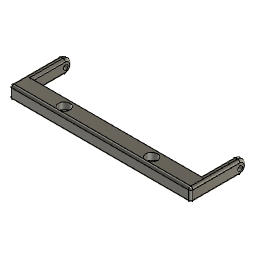
Q.R 2.0 A (Autodesk Fusion 360 design; units mm, degrees)
Autodesk Fusion 360 part; units mm, degrees
note: some values were not read from the file. Chosen so that the rebuilt part matches the saved one: which face or edge a step refers to. Set by a fixed rule: which sketch regions a step uses.
sketch "Sketch5" plane through (0, 0, -8) normal (0, 0, -1) x (1, 0, 0) in component "Arm 2.0 v7"
  arc A0 (69.5, 1.75) -> (68.5, 2.75) centre (68.5, 1.75) ccw
  line L0 (68.5, 2.75) -> (-0.75, 2.75)
  arc A1 (-0.75, 2.75) -> (-2.75, 0.75) centre (-0.75, 0.75) ccw
  line L1 (-2.75, 0.75) -> (-2.75, -47.25)
  arc A2 (-2.75, -47.25) -> (-0.75, -49.25) centre (-0.75, -47.25) ccw
  line L2 (-0.75, -49.25) -> (68.5, -49.25)
  arc A3 (68.5, -49.25) -> (69.5, -48.25) centre (68.5, -48.25) ccw
  line L3 (69.5, -48.25) -> (-1.75, -48.25)
  line L4 (-1.75, -48.25) -> (-1.75, 1.75)
  line L5 (-1.75, 1.75) -> (69.5, 1.75)
  line L6 (0.6613, 2.75) -> (-4.5, 2.75)
  line L7 (-2.75, -0.7377) -> (-2.75, 4.5)
  line L8 (-2.75, 2.75) -> (69.5271, 2.75)
  line L9 (69.5271, 2.75) -> (69.5271, -49.2656)
  line L10 (69.5271, -49.2656) -> (-2.75, -49.2656)
  line L11 (-2.75, -49.2656) -> (-2.75, 2.75)
  line L12 (70.0271, -49.7656) -> (-3.25, -49.7656)
  line L13 (-3.25, -49.7656) -> (-3.25, 3.25)
  line L14 (-3.25, 3.25) -> (70.0271, 3.25)
  line L15 (70.0271, 3.25) -> (70.0271, -49.7656)
  line L16 (73.0271, -52.7656) -> (-6.25, -52.7656)
  line L17 (-6.25, -52.7656) -> (-6.25, 6.25)
  line L18 (-6.25, 6.25) -> (73.0271, 6.25)
  line L19 (73.0271, 6.25) -> (73.0271, -52.7656)
  line L20 (79.5271, -59.2656) -> (-12.75, -59.2656)
  line L21 (-12.75, -59.2656) -> (-12.75, 12.75)
  line L22 (-12.75, 12.75) -> (79.5271, 12.75)
  line L23 (79.5271, 12.75) -> (79.5271, -59.2656)
  line L24 (82.5271, -62.2656) -> (-15.75, -62.2656)
  line L25 (-15.75, -62.2656) -> (-15.75, 15.75)
  line L26 (-15.75, 15.75) -> (82.5271, 15.75)
  line L27 (82.5271, 15.75) -> (82.5271, -62.2656)
  line L28 (-15.75, -3.25) -> (82.5271, -3.25)
  line L29 (-6.25, -3.25) -> (-6.25, 15.75)
  line L30 (70.0271, 3.25) -> (70.0271, 15.75)
  line L31 (73.0271, 6.25) -> (73.0271, 12.75)
  line L32 (-3.25, 3.25) -> (-3.25, 12.75)
  line L33 (73.0271, 12.75) -> (73.0271, 15.75)
  dimension "d13" = -0.5
  dimension "d14" = -3.5
  dimension "d15" = -10
  dimension "d16" = -13
  dimension "d17" = 6
  constraint coincident L0 L6.start
  constraint coincident L1 L7.start
  constraint perpendicular L6 L7
  constraint horizontal L8
  constraint vertical L9
  constraint horizontal L10
  constraint vertical L11
  constraint coincident L7 L8.start
  constraint coincident L6 L8.start
  constraint coincident L25 L28.start
  constraint coincident L27 L28.end
  constraint perpendicular L27 L28
  constraint coincident L17 L29.start
  constraint coincident L28 L29.start
  constraint coincident L26 L29.end
  constraint perpendicular L26 L29
  constraint coincident L26 L30.end
  constraint perpendicular L26 L30
  constraint coincident L22 L31.end
  constraint perpendicular L22 L31
  constraint coincident L22 L32.end
  constraint perpendicular L22 L32
  constraint coincident L26 L33.end
  constraint perpendicular L26 L33
  measures "d17" distance of L8 L28
extrude "Extrude2" add sketch "Sketch5" against normal blind 6 from surface at -2 contours L15 L18 L19 L28 L30 | L13 L17 L18 L28 L29 L32 | L18 L22 L30 L31 | L18 L22 L29 L32 | L22 L26 L30 L33 | L22 L26 L29 L30 in component "Arm 2.0 v7"
sketch "Sketch6" plane through (-6.25, 0, 0) normal (-1, 0, 0) x (0, -1, 0) in component "Arm 2.0 v7"
  line L0 (15.75, 0) -> (-3.25, 0)
  line L1 (-3.25, 0) -> (-3.25, -6)
  line L2 (-3.25, -6) -> (15.75, -6)
  line L3 (-3.25, -6) -> (2.3875, -0.3625)
  line L4 (-3.25, -6) -> (4.7226, -6) construction
  circle A0 centre (-0.4313, -3.1813) radius 1.05
  line L5 (15.75, -6) -> (15.75, 0)
  dimension "d23" = 45
  dimension "d24" = 2.1
  constraint horizontal L4
  constraint coincident L1.end L2.start
  constraint midpoint L3 A0.centre
  measures "d23" angle of L3 L4
  measures "d24" diameter of A0
extrude "Extrude3" cut sketch "Sketch6" against normal blind 85 contours L3 A0 | L3 A0 in component "Arm 2.0 v7"
fillet "Fillet2" [suppressed] in component "Arm 2.0 v7"
fillet "Fillet3" [suppressed] in component "Arm 2.0 v7"
extrude "Extrude4" add 1 faces at (20.1757, -15.75, -2) along direction (0, -1, 0) blind 6 in component "Arm 2.0 v7"
extrude "Extrude5" cut 1 faces at (21.1757, -12.75, -4) along direction (0, -1, 0) blind 2 in component "Arm 2.0 v7"
chamfer "Chamfer1" distance 2 distance2 6 1 edges at (33.3886, -14.75, -6) measured on face at (21.1757, -19.4167, -6) in component "Arm 2.0 v7"
sketch "Sketch1" plane through (0, 0, 0) normal (0, 0, 1) x (-1, 0, 0)
  line L0 (-70.0271, -3.25) -> (-70.0271, 14.75)
  line L1 (-70.0271, 14.75) -> (3.25, 14.75)
  line L2 (3.25, 14.75) -> (3.25, -3.25)
  line L3 (3.25, -3.25) -> (6.25, -3.25)
  line L4 (6.25, -3.25) -> (6.25, 21.75)
  line L5 (6.25, 21.75) -> (-73.0271, 21.75)
  line L6 (-73.0271, 21.75) -> (-73.0271, -3.25)
  line L7 (-73.0271, -3.25) -> (-70.0271, -3.25)
  line L8 (6.25, 21.75) -> (-73.0271, 21.75)
  line L9 (-73.0271, 21.75) -> (-73.0271, 14.75)
  line L10 (-73.0271, 14.75) -> (6.25, 14.75)
  line L11 (6.25, 14.75) -> (6.25, 21.75)
  line L12 (6.25, 18.25) -> (-73.0271, 18.25)
  circle A0 centre (-13.75, 18.25) radius 2.6
  circle A1 centre (-53.0271, 18.25) radius 2.6
  dimension "d7" = 7
  dimension "d8" = 5.2
  dimension "d9" = 5.2
  dimension "d10" = 20
  dimension "d11" = 20
  constraint horizontal L8
  constraint vertical L9
  constraint horizontal L10
  constraint vertical L11
  constraint coincident L6 L9.end
  constraint coincident L4.end L5.start
  constraint midpoint L11 L12.start
  constraint midpoint L9 L12.end
  constraint coincident L12 A0.centre
  constraint coincident L12 A1.centre
  measures "d7" distance of L4.end L10.end
  measures "d8" diameter of A0
  measures "d9" diameter of A1
  measures "d10" distance of L11 A0.centre
  measures "d11" distance of L9 A1.centre
extrude "Extrude6" cut sketch "Sketch1" against normal blind 3 contours L12 A1 | L12 A1 | L12 A0 | L12 A0 in component "Arm 2.0 v7"
extrude "Extrude7" add 1 faces at (-6.25, -14.7062, -3.0604) along direction (-1, 0, 0) blind 1 in component "Arm 2.0 v7"
extrude "Extrude8" cut 1 faces at (-3.25, -10.6906, -3.164) along direction (-1, 0, 0) blind 1 in component "Arm 2.0 v7"
extrude "Extrude9" add 1 faces at (73.0271, -14.7062, -3.0604) along direction (1, 0, 0) blind 1 in component "Arm 2.0 v7"
extrude "Extrude10" cut 1 faces at (70.0271, -10.6906, -3.164) along direction (1, 0, 0) blind 1 in component "Arm 2.0 v7"
fillet "Fillet5" radius 3 4 edges at (71.5271, 3.25, 0) (71.5271, 3.25, -6) (-4.75, 3.25, 0) (-4.75, 3.25, -6) in component "Arm 2.0 v7"
fillet "Fillet6" radius 1 2 edges at (33.3886, -21.75, -6) (33.3886, -21.75, 0) in component "Arm 2.0 v7"
fillet "Fillet8" radius 1 18 edges at (71.0271, -8.25, -6) (71.0271, 3.25, -3) (71.0271, -7.25, 0) (74.0271, -21.4571, -0.2929) (74.0271, -21.75, -3) (74.0271, -21.4571, -5.7071) (74.0271, -10.25, -6) (74.0271, 3.25, -3) (74.0271, -10.25, 0) (-7.25, -10.25, 0) (-7.25, -21.4571, -0.2929) (-7.25, -21.75, -3) (-7.25, -21.4571, -5.7071) (-7.25, -10.25, -6) (-7.25, 3.25, -3) (-4.25, -7.25, 0) (-4.25, 3.25, -3) (-4.25, -8.25, -6) in component "Arm 2.0 v7"
component "Arm 2.0 v7" placed x (1, 0, 0) y (0, 1, 0) z (0, 0, 1) at (0, 0, 0)
